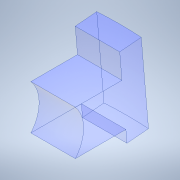
# Autodesk Inventor part: shank_2
Saved by Autodesk Inventor 2020.2 (Build 242310000, 310)
## iProperties
Created: 2021-01-30
Part Number: shank_2
Material: Generic
Document SubType Name: Modeling
Designer: DELL
Density: 1 g/cm^3
Appearance: Clear - Blue
Author: DELL
Autodesk Inventor part; units mm, degrees
ref_plane "XZ Plane" through (0, 0, 0) normal (0, 1, 0) x (-1, 0, 0)
ref_plane "XY Plane" through (0, 0, 0) normal (0, 0, 1) x (1, 0, 0)
ref_plane "UCS1: YZ Plane" through (0, 0, 0) normal (1, 0, 0) x (0, 1, 0)
sketch "Sketch20" plane through (0, 0, 0) normal (1, 0, 0) x (0, 1, 0)
  line L0 (-69.6588, 0) -> (90.205, 0) projected
  line L1 (0, -170.437) -> (0, 82.0728) construction
  circle A0 centre (0, 0) radius 40
  circle A1 centre (0, 0) radius 46
  line L2 (30, -34.8712) -> (30, -97.7573)
  line L3 (-30, -103.0066) -> (-30, -34.8712)
  line L4 (64.7527, -94.7169) -> (-46.8212, -104.4783)
  line L5 (64.7527, -94.7169) -> (67.3673, -124.6027)
  line L6 (67.3673, -124.6027) -> (-44.2065, -134.3641)
  line L7 (-44.2065, -134.3641) -> (-46.8212, -104.4783)
  point P0 (0, -100.382)
  dimension "d254" = 92
  dimension "d255" = 80
  dimension "d256" = 60
  dimension "d261" = 85
  dimension "d262" = 30
  dimension "d263" = 65
  dimension "d264" = 47
  dimension "d265" = 130
  dimension "d268" = 16.8854
  dimension "d269" = 34.8854
  constraints: 12 end point, 4 point on line, 2 centre point, 2 coincident, 2 parallel, 2 point on circle, 1 perpendicular, 1 vertical, 1 other
  measures "d254" diameter of A1
  measures "d255" diameter of A0
  measures "d256" distance between parallel lines of L2 L3
  measures "d261" angle of L1 L4
  measures "d262" distance of L4.start L5.end
  measures "d263" distance of L4.start point (0, -100.382)
  measures "d264" distance of L4.end point (0, -100.382)
  measures "d265" distance from line of L6 point (0, 0)
  measures "d268" distance of L4.end L3.start
  measures "d269" distance of L4.start L2.end
extrude "Extrusion18" add sketch "Sketch20" along normal mid plane 60 contours L2 L4 L3 A1 | L4 L5 L6 L7
sketch "Sketch21" plane through (-30, 64.7527, -94.7169) normal (0, 0.9961947, 0.0871557) x (1, 0, 0)
  line L0 (0, 0) -> (60, 0) projected
  line L1 (60, 30) -> (60, 0) projected
  line L2 (0, 30) -> (60, 30) projected
  line L3 (0, 0) -> (0, 30) projected
  line L4 (60, 30) -> (60, 0) projected
  line L5 (0, 0) -> (0, 30) projected
  arc A0 (60, 29.0992) -> (0, 29.0992) centre (30, -470) ccw
  line L6 (0, 30) -> (60, 30) projected
  point P0 (30, 30)
  point P1 (60, 29.0992)
  point P2 (0, 29.0992)
  dimension "d270" = 500
  constraints: 2 point on circle, 2 point on line, 1 centre point, 1 horizontal alignment, 1 tangent
  measures "d270" radius of A0
sketch3d "3D Sketch1"
  line L0 (-30, 67.3673, -124.6027) -> (-30, -44.2065, -134.3641)
  dimension "d173" = 92
  dimension "d174" = 80
  dimension "d224" = 60
  dimension "d230" = 2000
  dimension "d231" = 29.9943
  dimension "d233" = 10
  dimension "d235" = 2000
  dimension "d241" = 30
  dimension "d246" = 47
  dimension "d247" = 72
  dimension "d248" = 10
  dimension "d249" = 130
  dimension "d251" = 16.2947
  dimension "d252" = 40.92
sweep "Sweep1" cut profiles "Sketch21" path "3D Sketch1" keep normal constant yes contours L3 L2 A0 | A0 L2 L1
body "Solid1"
body "Solid8"
body "Solid9"
